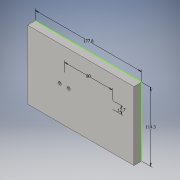
# Autodesk Inventor part: LoadCellLowerSide
Saved by Autodesk Inventor 2016 (Build 200138000, 138)
## iProperties
Created: 2018-12-06
Part Number: LoadCellLowerSide
Material: Generic
Document SubType Name: Modeling
Designer: Student
Density: 1 g/cm^3
Appearance: Default
Author: Student
Autodesk Inventor part; units mm, degrees
ref_plane "YZ Plane" through (0, 0, 0) normal (1, 0, 0) x (0, 1, 0)
ref_plane "XZ Plane" through (0, 0, 0) normal (0, 1, 0) x (-1, 0, 0)
ref_plane "XY Plane" through (0, 0, 0) normal (0, 0, 1) x (1, 0, 0)
sketch "Sketch1" plane through (0, 0, 0) normal (0, 0, 1) x (1, 0, 0)
  line L0 (-88.9, -57.15) -> (88.9, -57.15)
  line L1 (88.9, -57.15) -> (88.9, 57.15)
  line L2 (88.9, 57.15) -> (-88.9, 57.15)
  line L3 (-88.9, 57.15) -> (-88.9, -57.15)
  line L4 (-40, -6.35) -> (40, -6.35)
  line L5 (40, -6.35) -> (40, 6.35)
  line L6 (40, 6.35) -> (-40, 6.35)
  line L7 (-40, 6.35) -> (-40, -6.35)
  point P0 (-35, 0)
  point P1 (-20, 0)
  dimension "d0" = 177.8
  dimension "d1" = 114.3
  dimension "d2" = 80
  dimension "d3" = 12.7
  constraints: 16 end point, 4 parallel, 2 horizontal, 2 perpendicular
  measures "d0" distance of L2.end L1.end
  measures "d1" distance of L1.end L0.end
  measures "d2" distance of L6.end L5.end
  measures "d3" distance of L5.end L4.end
extrude "Extrusion1" add sketch "Sketch1" along normal blind 12.7 contours L3 L2 L1 L0 | L7 L6 L5 L4
hole "Hole1" at (-35, 0, 0) at (-20, 0, 0) direction (0, 0, 1) diameter 5 end through all
body "Solid1"
